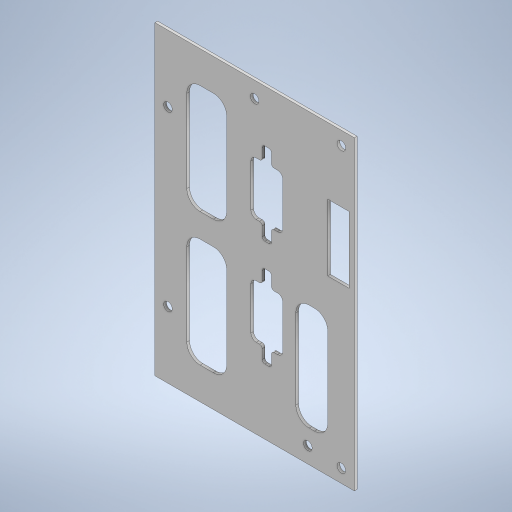
# Autodesk Inventor part: front
Saved by Autodesk Inventor 2023 (Build 270158000, 158)
## iProperties
Created: 2023-05-25
Part Number: front
Material: 一般
Document SubType Name: Sheet Metal
Designer: 310611102
Density: 1 g/cm^3
Sheet Metal Rule: Default_mm
Appearance: 預設
Author: 310611102
Autodesk Inventor part; units mm, degrees
ref_plane "YZ Plane" through (0, 0, 0) normal (1, 0, 0) x (0, 1, 0)
ref_plane "XZ Plane" through (0, 0, 0) normal (0, 1, 0) x (-1, 0, 0)
ref_plane "XY Plane" through (0, 0, 0) normal (0, 0, 1) x (1, 0, 0)
sketch "Sketch1" plane through (0, 0, 0) normal (0, 0, 1) x (1, 0, 0)
  line L0 (-37.5, 57.5) -> (37.5, 57.5)
  line L1 (37.5, 57.5) -> (37.5, -57.5)
  line L2 (37.5, -57.5) -> (-37.5, -57.5)
  line L3 (-37.5, -57.5) -> (-37.5, 57.5)
  line L4 (-37.5, 57.5) -> (37.5, -57.5) construction
  line L5 (37.5, 57.5) -> (-37.5, -57.5) construction
  line L6 (0, 0) -> (0, 12.9993)
  circle A0 centre (-32.6, -32.5) radius 1.6
  circle A1 centre (0, 51.5) radius 1.6
  line L7 (0, 0) -> (8.7382, 0)
  circle A2 centre (20, -51.5) radius 1.6
  circle A3 centre (-32.6, 32.5) radius 1.6
  circle A4 centre (32.6, 52.5) radius 1.6
  circle A5 centre (32.6, -52.5) radius 1.6
  line L8 (10.6, -9.5) -> (10.6, -25.5)
  line L9 (-1.4, -25.5) -> (-1.4, -9.5)
  line L10 (-1.4, -7.5) -> (10.6, -27.5) construction
  line L11 (10.6, -7.5) -> (-1.4, -27.5) construction
  line L12 (3.85, -2) -> (5.35, -2)
  line L13 (6.35, -3) -> (6.35, -6.5)
  line L14 (2.85, -6.5) -> (2.85, -3)
  line L15 (2.85, -2) -> (6.35, -7.5) construction
  line L16 (6.35, -2) -> (2.85, -7.5) construction
  line L17 (3.85, -33) -> (5.35, -33)
  line L18 (6.35, -32) -> (6.35, -28.5)
  line L19 (2.85, -28.5) -> (2.85, -32)
  line L20 (2.85, -33) -> (6.35, -27.5) construction
  line L21 (6.35, -33) -> (2.85, -27.5) construction
  line L22 (35.5, 7.5) -> (27.5, 7.5)
  line L23 (27.5, 7.5) -> (27.5, 32.5)
  line L24 (27.5, 32.5) -> (35.5, 32.5)
  line L25 (35.5, 32.5) -> (35.5, 7.5)
  line L26 (35.5, 7.5) -> (27.5, 32.5) construction
  line L27 (27.5, 7.5) -> (35.5, 32.5) construction
  line L28 (-15.5, -45.5) -> (-20.5, -45.5)
  line L29 (-25.5, -40.5) -> (-25.5, -9.5)
  line L30 (-20.5, -4.5) -> (-15.5, -4.5)
  line L31 (-10.5, -9.5) -> (-10.5, -40.5)
  line L32 (-10.5, -45.5) -> (-25.5, -4.5) construction
  line L33 (-25.5, -45.5) -> (-10.5, -4.5) construction
  arc A6 (-15.5, -45.5) -> (-10.5, -40.5) centre (-15.5, -40.5) ccw
  arc A7 (-10.5, -9.5) -> (-15.5, -4.5) centre (-15.5, -9.5) ccw
  arc A8 (-20.5, -4.5) -> (-25.5, -9.5) centre (-20.5, -9.5) ccw
  arc A9 (-25.5, -40.5) -> (-20.5, -45.5) centre (-20.5, -40.5) ccw
  line L34 (-15.5, 45.5) -> (-20.5, 45.5)
  line L35 (-25.5, 40.5) -> (-25.5, 9.5)
  line L36 (-20.5, 4.5) -> (-15.5, 4.5)
  line L37 (-10.5, 9.5) -> (-10.5, 40.5)
  line L38 (-10.5, 45.5) -> (-25.5, 4.5) construction
  line L39 (-25.5, 45.5) -> (-10.5, 4.5) construction
  arc A10 (-10.5, 40.5) -> (-15.5, 45.5) centre (-15.5, 40.5) ccw
  arc A11 (-15.5, 4.5) -> (-10.5, 9.5) centre (-15.5, 9.5) ccw
  arc A12 (-25.5, 9.5) -> (-20.5, 4.5) centre (-20.5, 9.5) ccw
  arc A13 (-20.5, 45.5) -> (-25.5, 40.5) centre (-20.5, 40.5) ccw
  line L40 (22.5, -45.5) -> (20.5, -45.5)
  line L41 (15.5, -40.5) -> (15.5, -10.5)
  line L42 (20.5, -5.5) -> (22.5, -5.5)
  line L43 (27.5, -10.5) -> (27.5, -40.5)
  line L44 (27.5, -45.5) -> (15.5, -5.5) construction
  line L45 (15.5, -45.5) -> (27.5, -5.5) construction
  arc A14 (22.5, -45.5) -> (27.5, -40.5) centre (22.5, -40.5) ccw
  arc A15 (15.5, -40.5) -> (20.5, -45.5) centre (20.5, -40.5) ccw
  arc A16 (27.5, -10.5) -> (22.5, -5.5) centre (22.5, -10.5) ccw
  arc A17 (20.5, -5.5) -> (15.5, -10.5) centre (20.5, -10.5) ccw
  arc A18 (2.85, -32) -> (3.85, -33) centre (3.85, -32) ccw
  arc A19 (5.35, -33) -> (6.35, -32) centre (5.35, -32) ccw
  arc A20 (6.35, -3) -> (5.35, -2) centre (5.35, -3) ccw
  arc A21 (3.85, -2) -> (2.85, -3) centre (3.85, -3) ccw
  line L46 (0.6, -7.5) -> (1.85, -7.5)
  line L47 (7.35, -7.5) -> (8.6, -7.5)
  line L48 (8.6, -27.5) -> (7.35, -27.5)
  line L49 (1.85, -27.5) -> (0.6, -27.5)
  arc A22 (8.6, -27.5) -> (10.6, -25.5) centre (8.6, -25.5) ccw
  arc A23 (10.6, -9.5) -> (8.6, -7.5) centre (8.6, -9.5) ccw
  arc A24 (-1.4, -25.5) -> (0.6, -27.5) centre (0.6, -25.5) ccw
  arc A25 (0.6, -7.5) -> (-1.4, -9.5) centre (0.6, -9.5) ccw
  arc A26 (2.85, -28.5) -> (1.85, -27.5) centre (1.85, -28.5) ccw
  arc A27 (7.35, -27.5) -> (6.35, -28.5) centre (7.35, -28.5) ccw
  arc A28 (6.35, -6.5) -> (7.35, -7.5) centre (7.35, -6.5) ccw
  arc A29 (1.85, -7.5) -> (2.85, -6.5) centre (1.85, -6.5) ccw
  line L50 (2.85, 11.5) -> (2.85, 8)
  arc A30 (7.35, 12.5) -> (6.35, 11.5) centre (7.35, 11.5) ccw
  arc A31 (8.6, 12.5) -> (10.6, 14.5) centre (8.6, 14.5) ccw
  line L51 (8.6, 12.5) -> (7.35, 12.5)
  arc A32 (2.85, 8) -> (3.85, 7) centre (3.85, 8) ccw
  line L52 (2.85, 7) -> (6.35, 12.5) construction
  line L53 (6.35, 7) -> (2.85, 12.5) construction
  line L54 (6.35, 8) -> (6.35, 11.5)
  line L55 (3.85, 7) -> (5.35, 7)
  arc A33 (5.35, 7) -> (6.35, 8) centre (5.35, 8) ccw
  line L56 (-1.4, 14.5) -> (-1.4, 30.5)
  arc A34 (2.85, 11.5) -> (1.85, 12.5) centre (1.85, 11.5) ccw
  line L57 (1.85, 12.5) -> (0.6, 12.5)
  arc A35 (-1.4, 14.5) -> (0.6, 12.5) centre (0.6, 14.5) ccw
  line L58 (7.35, 32.5) -> (8.6, 32.5)
  arc A36 (10.6, 30.5) -> (8.6, 32.5) centre (8.6, 30.5) ccw
  line L59 (3.85, 38) -> (5.35, 38)
  line L60 (6.35, 37) -> (6.35, 33.5)
  line L61 (2.85, 33.5) -> (2.85, 37)
  line L62 (2.85, 38) -> (6.35, 32.5) construction
  line L63 (6.35, 38) -> (2.85, 32.5) construction
  line L64 (0.6, 32.5) -> (1.85, 32.5)
  arc A37 (1.85, 32.5) -> (2.85, 33.5) centre (1.85, 33.5) ccw
  arc A38 (0.6, 32.5) -> (-1.4, 30.5) centre (0.6, 30.5) ccw
  arc A39 (3.85, 38) -> (2.85, 37) centre (3.85, 37) ccw
  arc A40 (6.35, 37) -> (5.35, 38) centre (5.35, 37) ccw
  arc A41 (6.35, 33.5) -> (7.35, 32.5) centre (7.35, 33.5) ccw
  line L65 (10.6, 30.5) -> (10.6, 14.5)
  line L66 (-1.4, 32.5) -> (10.6, 12.5) construction
  line L67 (10.6, 32.5) -> (-1.4, 12.5) construction
  point P0 (4.6, -17.5)
  point P1 (4.6, -4.75)
  point P2 (4.6, -30.25)
  point P3 (31.5, 20)
  point P4 (-18, -25)
  point P5 (-18, 25)
  point P6 (21.5, -25.5)
  point P7 (4.6, 9.75)
  point P8 (4.6, 35.25)
  point P9 (4.6, 22.5)
  point P10 (0, 57.5)
  point P11 (0, -57.5)
  dimension "d0" = 115
  dimension "d1" = 75
  dimension "d22" = 3.2
  dimension "d25" = 3.2
  dimension "d26" = 6
  dimension "d27" = 25
  dimension "d28" = 4.9
  dimension "d29" = 3.2
  dimension "d30" = 4.9
  dimension "d31" = 5
  dimension "d32" = 5.5
  dimension "d33" = 3.5
  dimension "d34" = 12
  dimension "d35" = 20
  dimension "d38" = 36.1
  dimension "d39" = 8
  dimension "d40" = 25
  dimension "d41" = 2
  dimension "d42" = 25
  dimension "d43" = 41
  dimension "d44" = 15
  dimension "d45" = 12
  dimension "d46" = 12
  dimension "d47" = 5
  dimension "d48" = 40
  dimension "d49" = 12
  dimension "d50" = 10
  dimension "d51" = 12
  dimension "d52" = 5
  dimension "d53" = 1
  dimension "d54" = 30
  dimension "d55" = 2
  dimension "d56" = 1
  dimension "d59" = 40
  dimension "d64" = 9
  dimension "d65" = 12
  dimension "d67" = 0
  dimension "d68" = 3.2
  dimension "d69" = 6
  dimension "d70" = 20
  measures "d0" distance of L0.end L1.end
  measures "d1" distance of L0.start L0.end
  measures "d22" diameter of A0
  measures "d25" diameter of A1
  measures "d26" distance from line of L0 A1.centre
  measures "d27" distance from line of L2 A0.centre
  measures "d28" distance from line of L3 A0.centre
  measures "d29" diameter of A4
  measures "d30" distance from line of L1 A4.centre
  measures "d31" distance from line of L0 A4.centre
  measures "d32" distance of L15.end L16.start
  measures "d33" distance of L15.start L16.start
  measures "d34" distance of L10.start L11.start
  measures "d35" distance of L11.start L10.end
  measures "d38" distance between parallel lines of L3 L9
  measures "d39" distance of L23.end L24.end
  measures "d40" distance of L24.end L22.start
  measures "d41" distance between parallel lines of L1 L25
  measures "d42" distance between parallel lines of L0 L24
  measures "d43" distance of L33.start L32.end
  measures "d44" distance of L32.start L33.start
  measures "d45" distance between parallel lines of L3 L29
  measures "d46" distance between parallel lines of L2 L28
  measures "d47" radius of A6
  measures "d48" distance of L45.end L44.start
  measures "d49" distance of L44.end L45.end
  measures "d50" distance between parallel lines of L1 L43
  measures "d51" distance between parallel lines of L2 L40
  measures "d52" radius of A14
  measures "d53" radius of A18
  measures "d54" distance between parallel lines of L2 L48
  measures "d55" radius of A22
  measures "d56" radius of A26
  measures "d59" distance of L10.end L66.end
  measures "d64" distance between parallel lines of L36 L30
  measures "d65" distance between parallel lines of L0 L34
  measures "d67" horizontal distance of point (0, 57.5) A1.centre
  measures "d68" diameter of A2
  measures "d69" distance from line of L2 A2.centre
  measures "d70" horizontal distance of point (0, -57.5) A2.centre
extrude "Plate1" add sketch "Sketch1" along normal blind 1
equation "\"d2\" = 厚度"
equation "\"折彎半徑\" = 厚度"
equation "\"折彎離隙寬度\" = 厚度"
equation "\"折彎離隙深度\" = 0.5 * 厚度"
equation "\"轉角離隙大小\" = 4 * 厚度"
equation "\"最小剩餘\" = 2 * 厚度"
equation "\"轉移半徑\" = 折彎半徑"
equation "\"Jacobi半徑大小\" = 折彎半徑"
equation "\"間隙大小\" = 厚度"
equation "\"厚度\" = 1"
body "Solid1"
